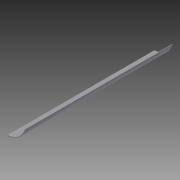
# Autodesk Inventor part: Scoop
Saved by Autodesk Inventor 2015 (Build 190159000, 159)
## iProperties
Created: 2015-10-02
Part Number: Scoop
Material: Generic
Document SubType Name: Modeling
Designer: damedin
Density: 1 g/cm^3
Appearance: Default
Author: damedin
Autodesk Inventor part; units mm, degrees
ref_plane "YZ Plane" through (0, 0, 0) normal (1, 0, 0) x (0, 1, 0)
ref_plane "XZ Plane" through (0, 0, 0) normal (0, 1, 0) x (-1, 0, 0)
ref_plane "XY Plane" through (0, 0, 0) normal (0, 0, 1) x (1, 0, 0)
sketch "Sketch1" plane through (0, 0, 0) normal (0, 0, 1) x (1, 0, 0)
  arc A0 (-10.8182, -7.0955) -> (8.9091, 8.8137) centre (-11.7385, 14.2312) ccw
  line L0 (-10.8182, -7.0955) -> (-10.8182, -6.5729)
  line L1 (8.9091, 8.8137) -> (8.3707, 8.8137)
  arc A1 (-10.8182, -6.5729) -> (8.3707, 8.8137) centre (-11.5148, 13.9547) ccw
  point P0 (0, 0)
  constraints: 4 end point, 4 point on circle, 2 centre point, 1 horizontal, 1 vertical
extrude "Extrusion1" add sketch "Sketch1" along normal blind 159.9946
body "Solid1"
